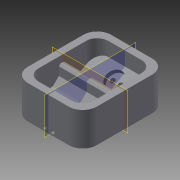
# Autodesk Inventor part: Line Tracker v3
Saved by Autodesk Inventor 2015 (Build 190159000, 159)
## iProperties
Created: 2015-04-19
Part Number: Line Tracker v3
Material: Generic
Document SubType Name: Modeling
Designer: Kyle
Density: 1 g/cm^3
Appearance: Default
Author: Kyle
Autodesk Inventor part; units mm, degrees
ref_plane "YZ Plane" through (0, 0, 0) normal (1, 0, 0) x (0, 1, 0)
ref_plane "XZ Plane" through (0, 0, 0) normal (0, 1, 0) x (-1, 0, 0)
ref_plane "XY Plane" through (0, 0, 0) normal (0, 0, 1) x (1, 0, 0)
sketch "Sketch1" plane through (0, 0, 0) normal (1, 0, 0) x (0, 1, 0)
  line L0 (0, 0) -> (0, 9.525)
  line L1 (0, 9.525) -> (7.62, 9.525)
  line L2 (7.62, 9.525) -> (7.62, 8.001)
  line L3 (7.62, 8.001) -> (4.445, 8.001)
  line L4 (4.445, 8.001) -> (1.56, 3.004)
  line L5 (3.8019, 0.762) -> (6.0879, 0.762)
  line L6 (6.0879, 0.762) -> (6.0879, 0)
  line L7 (0, 0) -> (6.0879, 0) construction
  line L8 (1.56, 3.004) -> (3.8019, 0.762)
  line L9 (0, 0) -> (0, -9.525)
  line L10 (0, -9.525) -> (7.62, -9.525)
  line L11 (7.62, -9.525) -> (7.62, -8.001)
  line L12 (7.62, -8.001) -> (4.445, -8.001)
  line L13 (4.445, -8.001) -> (1.56, -3.004)
  line L14 (3.8019, -0.762) -> (6.0879, -0.762)
  line L15 (6.0879, -0.762) -> (6.0879, 0)
  line L16 (1.56, -3.004) -> (3.8019, -0.762)
  dimension "d0" = 9.525
  dimension "d1" = 120
  dimension "d2" = 1.524
  dimension "d3" = 7.62
  dimension "d6" = 135
  dimension "d7" = 2.286
  dimension "d8" = 0.762
  dimension "d9" = 3.175
  constraints: 34 end point, 7 symmetric about line, 4 perpendicular, 2 horizontal, 1 vertical
  measures "d0" distance of L0.start L0.end
  measures "d1" angle of L4 L3
  measures "d2" distance of L1.end L2.end
  measures "d3" distance of L0.end L1.end
  measures "d6" angle of L5 L8
  measures "d7" distance of L5.start L5.end
  measures "d8" distance of L5.end L6.end
  measures "d9" distance of L2.end L3.end
extrude "Extrusion1" add sketch "Sketch1" along normal mid plane 12.7
sketch "Sketch2" plane through (6.35, 0, 0) normal (1, 0, 0) x (0, 0, -1)
  line L0 (-9.518, 7.6231) -> (9.525, 7.6231)
  line L1 (9.525, 7.6231) -> (9.525, 0)
  line L2 (9.525, 0) -> (-9.518, 0)
  line L3 (-9.518, 0) -> (-9.518, 7.6231)
  point P0 (0, 0)
  constraints: 8 end point, 2 parallel, 1 horizontal, 1 perpendicular
extrude "Extrusion2" add sketch "Sketch2" along normal blind 1.524
ref_plane "Work Plane1" through (0, 0, 0) normal (-1, 0, 0) x (0, 0, 1)
mirror "Mirror1" about plane through (0, 0, 0) normal (-1, 0, 0) of "Extrusion2"
ref_plane "Work Plane2" through (6.35, 4.445, 0) normal (0, 0, 1) x (1, 0, 0)
sketch "Sketch3" plane through (-6.35, 1.56, -3.004) normal (0, 0.8660254, 0.5) x (1, 0, 0)
  circle A0 centre (6.35, 2.9685) radius 1.905
  line L0 (6.35, -3.3815) -> (6.35, 2.9685) construction
  line L1 (12.7, 0.3224) -> (0, 0.3224) construction
  dimension "d14" = 3.81
  dimension "d15" = 6.35
  constraints: 2 end point, 1 centre point, 1 perpendicular
  measures "d14" diameter of A0
  measures "d15" distance of L0.start L0.end
extrude "Extrusion3" cut sketch "Sketch3" against normal blind 1.016
mirror "Mirror2" about plane through (6.35, 4.445, 0) normal (0, 0, 1) of "Extrusion3"
sketch "Sketch4" plane through (0, 2.1643, 6.0828) normal (0, 0.8660254, -0.5) x (1, 0, 0)
  line L0 (0, 0) -> (0.889, 0)
  circle A0 centre (0.889, 0) radius 0.508
  line L1 (0, 0) -> (0, -1.5045) construction
  line L2 (0, 0) -> (-0.889, 0)
  circle A1 centre (-0.889, 0) radius 0.508
  line L3 (-3.9808, -2.9089) -> (3.3924, -2.9089) construction
  point P0 (0, 6.35)
  dimension "d18" = 0.889
  dimension "d19" = 1.016
  constraints: 8 end point, 2 centre point, 2 coincident, 2 horizontal, 2 symmetric about line, 1 vertical, 1 other
  measures "d18" distance of L0.start L0.end
  measures "d19" diameter of A0
revolve "Revolution1" cut sketch "Sketch4" angle 90 about axis through (-3.9808, 3.6188, 8.602) along (-1, 0, 0)
mirror "Mirror3" about plane through (6.35, 4.445, 0) normal (0, 0, 1) of "Revolution1"
fillet "Fillet1" radius 3.175 6 edges at (-7.874, 3.8115, 9.518) (-6.35, 3.81, 9.525) (7.874, 3.8115, 9.518) (6.35, 3.81, 9.525) (7.874, 3.8115, -9.525) (-7.874, 3.8115, -9.525)
fillet "Fillet2" radius 2.54 4 edges at (-6.35, 6.0325, 8.001) (6.35, 6.0325, 8.001) (6.35, 6.0325, -8.001) (-6.35, 6.0325, -8.001)
chamfer "Chamfer1" distance 1.27 angle 45 2 edges at (0, 1.56, 3.004) (0, 1.56, -3.004)
chamfer "Chamfer2" distance 0.381 angle 45 2 edges at (0, 6.0879, -0.762) (0, 6.0879, 0.762)
body "Solid1"
